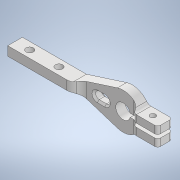
# Autodesk Inventor part: arm_1
Saved by Autodesk Inventor 2020 (Build 240168000, 168)
## iProperties
Created: 2020-01-20
Part Number: arm_1
Material: Generic
Document SubType Name: Modeling
Designer: psrobotics
Density: 1 g/cm^3
Appearance: Default
Author: psrobotics
Autodesk Inventor part; units mm, degrees
ref_plane "YZ Plane" through (0, 0, 0) normal (1, 0, 0) x (0, 1, 0)
ref_plane "XZ Plane" through (0, 0, 0) normal (0, 1, 0) x (-1, 0, 0)
ref_plane "XY Plane" through (0, 0, 0) normal (0, 0, 1) x (1, 0, 0)
sketch "Sketch1" plane through (0, 0, 0) normal (0, 0, 1) x (1, 0, 0)
  circle A0 centre (0, 0) radius 4 projected
  circle A1 centre (0, 0) radius 4
  line L0 (0, 0) -> (-60, 0)
  circle A2 centre (0, 0) radius 10
  line L1 (-60, 0) -> (-60, -2.5)
  line L2 (-60, -2.5) -> (-25, -2.5)
  line L3 (-25, -2.5) -> (-25, 2.5)
  line L4 (-25, 2.5) -> (-60, 2.5)
  line L5 (-60, 2.5) -> (-60, -2.5)
  line L6 (-25, -2.5) -> (-3.0476, -9.5243)
  line L7 (-25, 2.5) -> (-3.0476, 9.5243)
  point P0 (0, 0)
  dimension "d0" = 8
  dimension "d1" = 60
  dimension "d2" = 20
  dimension "d3" = 2.5
  dimension "d4" = 35
  dimension "d5" = 5
  constraints: 16 end point, 2 centre point, 2 coincident, 2 horizontal, 2 parallel, 2 point on circle, 2 tangent, 1 perpendicular, 1 vertical
  measures "d0" diameter of A1
  measures "d1" distance of L0.start L0.end
  measures "d2" diameter of A2
  measures "d3" distance of L0.end L1.end
  measures "d4" distance of L4.end L3.end
  measures "d5" distance of L3.end L2.end
extrude "Extrusion1" add sketch "Sketch1" against normal blind 5
sketch "Sketch2" plane through (0, 0, 0) normal (0, 0, 1) x (1, 0, 0)
  line L0 (-60, 2.5) -> (-60, -2.5) projected
  line L1 (-60, -2.5) -> (-25, -2.5) projected
  line L2 (-25, -2.5) -> (-3.0476, -9.5243) projected
  arc A0 (-3.0476, -9.5243) -> (-3.0476, 9.5243) centre (0, 0) ccw projected
  line L3 (-3.0476, 9.5243) -> (-25, 2.5) projected
  line L4 (-25, 2.5) -> (-60, 2.5) projected
  circle A1 centre (0, 0) radius 4 projected
  line L5 (0, 0) -> (7.6, 0)
  line L6 (13.6, -1) -> (13.6, 1)
  line L7 (13.6, 1) -> (1.6, 1)
  line L8 (1.6, 1) -> (1.6, -1)
  line L9 (1.6, -1) -> (13.6, -1)
  line L10 (13.6, -1) -> (1.6, 1) construction
  line L11 (13.6, 1) -> (1.6, -1) construction
  point P0 (0, 0)
  dimension "d8" = 7.6
  dimension "d9" = 2
  dimension "d10" = 12
  constraints: 14 end point, 2 midpoint, 2 parallel, 2 perpendicular, 1 horizontal
  measures "d8" distance of L5.start L5.end
  measures "d9" distance of L6.start L6.end
  measures "d10" distance of L7.end L6.end
extrude "Extrusion2" cut sketch "Sketch2" against normal blind 5 contours L7 L6 L9 A0 | A0 L9 A1 L7 | A1 L5 L8 L7 | L9 L8 L5 A1
sketch "Sketch3" plane through (0, 0, 0) normal (0, 0, 1) x (1, 0, 0)
  line L0 (3.873, 1) -> (9.9499, 1) projected
  arc A0 (9.9499, 1) -> (-3.0476, 9.5243) centre (0, 0) ccw projected
  line L1 (-3.0476, 9.5243) -> (-25, 2.5) projected
  line L2 (-25, 2.5) -> (-60, 2.5) projected
  line L3 (-60, 2.5) -> (-60, -2.5) projected
  line L4 (-60, -2.5) -> (-25, -2.5) projected
  line L5 (-25, -2.5) -> (-3.0476, -9.5243) projected
  arc A1 (-3.0476, -9.5243) -> (9.9499, -1) centre (0, 0) ccw projected
  line L6 (9.9499, -1) -> (3.873, -1) projected
  arc A2 (3.873, 1) -> (3.873, -1) centre (0, 0) ccw projected
  line L7 (3.873, -1) -> (21.873, -1)
  line L8 (21.873, -1) -> (21.873, -5)
  line L9 (21.873, -5) -> (3.873, -5)
  line L10 (3.873, -5) -> (3.873, -1)
  arc A3 (3.873, 1) -> (3.873, -1) centre (0, 0) ccw projected
  line L11 (3.873, 1) -> (21.873, 1)
  line L12 (21.873, 1) -> (21.873, 5)
  line L13 (21.873, 5) -> (3.873, 5)
  line L14 (3.873, 5) -> (3.873, 1)
  point P0 (0, 0)
  point P1 (9.9499, 1)
  point P2 (9.9499, -1)
  dimension "d13" = 18
  dimension "d14" = 4
  dimension "d15" = 18
  dimension "d16" = 4
  constraints: 16 end point, 4 parallel, 2 horizontal, 2 perpendicular
  measures "d13" distance of L8.end L9.end
  measures "d14" distance of L7.end L8.end
  measures "d15" distance of L13.end L12.end
  measures "d16" distance of L12.end L11.end
extrude "Extrusion3" add sketch "Sketch3" against normal blind 5 contours L14 L13 A0 L0 | A0 L13 L12 L11 | L6 A1 L9 L10 | L7 L8 L9 A1
sketch "Sketch4" plane through (8.6603, 5, 0) normal (0, 1, 0) x (1, 0, 0)
  line L0 (0, 0) -> (0, 5) projected
  line L1 (13.2127, 0) -> (0, 0) projected
  line L2 (13.2127, 0) -> (13.2127, 5) projected
  line L3 (0, 5) -> (13.2127, 5) projected
  line L4 (13.2127, 0) -> (13.2127, 5) projected
  line L5 (13.2127, 5) -> (0, 5)
  line L6 (0, 5) -> (0, -3)
  line L7 (0, -3) -> (13.2127, -3)
  line L8 (13.2127, -3) -> (13.2127, 5)
  point P0 (-8.6603, 0)
  dimension "d19" = 8
  constraints: 8 end point, 2 parallel, 1 horizontal, 1 perpendicular
  measures "d19" distance of L5.end L6.end
extrude "Extrusion4" add sketch "Sketch4" against normal blind 4 contours L1 L8 L7 L6
sketch "Sketch5" plane through (8.6603, -5, 0) normal (0, -1, 0) x (1, 0, 0)
  line L0 (0, 0) -> (0, -5) projected
  line L1 (0, 0) -> (0, 3) projected
  line L2 (0, 3) -> (13.2127, 3) projected
  line L3 (13.2127, 3) -> (13.2127, -5) projected
  line L4 (0, -5) -> (13.2127, -5) projected
  point P0 (-8.6603, 0)
extrude "Extrusion5" add sketch "Sketch5" against normal blind 4
sketch "Sketch6" plane through (8.6603, -5, -5) normal (0, -1, 0) x (1, 0, 0)
  line L0 (0, 0) -> (0, 5) projected
  line L1 (13.2127, 0) -> (0, 0) projected
  line L2 (13.2127, 0) -> (13.2127, 8) projected
  line L3 (13.2127, 8) -> (0, 8) projected
  line L4 (0, 8) -> (0, 5) projected
  line L5 (13.2127, 8) -> (13.2127, 0) projected
  line L6 (13.2127, 4) -> (6.6064, 4)
  circle A0 centre (6.6064, 4) radius 1.5
  point P0 (-8.6603, 5)
  dimension "d24" = 3
  constraints: 2 end point, 1 centre point, 1 coincident, 1 midpoint, 1 perpendicular
  measures "d24" diameter of A0
extrude "Extrusion6" cut sketch "Sketch6" against normal blind 10 contours A0
fillet "Fillet1" radius 3 2 edges at (8.6603, -3, 0) (8.6603, 3, 0)
sketch "Sketch7" plane through (-60, -2.5, 0) normal (0, -1, 0) x (1, 0, 0)
  line L0 (0, 0) -> (35, 0) projected
  line L1 (0, 0) -> (0, -5) projected
  line L2 (35, -5) -> (0, -5) projected
  line L3 (35, 0) -> (35, -5) projected
  line L4 (35, -5) -> (0, -5) projected
  line L5 (0, -5) -> (35, -5)
  line L6 (35, -5) -> (35, 3)
  line L7 (35, 3) -> (0, 3)
  line L8 (0, 3) -> (0, -5)
  point P0 (60, 0)
  dimension "d28" = 35
  dimension "d29" = 8
  constraints: 8 end point, 2 parallel, 1 horizontal, 1 perpendicular
  measures "d28" distance of L7.end L6.end
  measures "d29" distance of L6.end L5.end
extrude "Extrusion7" add sketch "Sketch7" against normal blind 5
fillet "Fillet2" radius 6 1 edges at (-25, 0, 0)
fillet "Fillet3" radius 1.5 4 edges at (21.873, -3, 3) (21.873, 3, 3) (21.873, -3, -5) (21.873, 3, -5)
fillet "Fillet4" radius 3 2 edges at (8.6603, 5, -1) (8.6603, -5, -1)
fillet "Fillet5" radius 2 2 edges at (8.6603, -3.227, 3) (8.6603, 3.227, 3)
sketch "Sketch8" plane through (0, 0, 0) normal (0, 0, 1) x (1, 0, 0)
  line L0 (-19.8038, -4.1627) -> (-19.8038, 4.1627) projected
  line L1 (-19.8038, -4.1627) -> (-3.0476, -9.5243) projected
  arc A0 (-3.0476, -9.5243) -> (5.6603, -8.2439) centre (0, 0) ccw projected
  line L2 (5.6603, -1) -> (5.6603, -8.2439) projected
  line L3 (5.6603, -1) -> (3.873, -1) projected
  arc A1 (3.873, 1) -> (3.873, -1) centre (0, 0) ccw projected
  line L4 (3.873, 1) -> (5.6603, 1) projected
  line L5 (5.6603, 8.2439) -> (5.6603, 1) projected
  arc A2 (5.6603, 8.2439) -> (-3.0476, 9.5243) centre (0, 0) ccw projected
  line L6 (-3.0476, 9.5243) -> (-19.8038, 4.1627) projected
  line L7 (0, 0) -> (-12, 0)
  line L8 (-10, 0) -> (-14, 0) construction
  line L9 (-10, 2) -> (-14, 2)
  line L10 (-14, -2) -> (-10, -2)
  arc A3 (-10, -2) -> (-10, 2) centre (-10, 0) ccw
  arc A4 (-14, 2) -> (-14, -2) centre (-14, 0) ccw
  point P0 (0, 0)
  dimension "d36" = 12
  dimension "d37" = 2
  dimension "d38" = 4
  constraints: 10 end point, 4 point on circle, 4 tangent, 2 centre point, 2 horizontal, 1 midpoint, 1 parallel
  measures "d36" distance of L7.start L7.end
  measures "d37" distance of L7.end L8.end
  measures "d38" diameter of A4
extrude "Extrusion8" cut sketch "Sketch8" against normal blind 5 contours A3 L10 A4 L9
sketch "Sketch9" plane through (-60, -2.5, -5) normal (0, -1, 0) x (1, 0, 0)
  line L0 (0, 8) -> (0, 0) projected
  line L1 (35, 0) -> (0, 0) projected
  line L2 (35, 0) -> (35, 8) projected
  line L3 (35, 8) -> (0, 8) projected
  line L4 (0, 8) -> (0, 0) projected
  line L5 (0, 4) -> (8, 4)
  line L6 (8, 4) -> (24, 4)
  circle A0 centre (24, 4) radius 2
  circle A1 centre (8, 4) radius 2
  point P0 (60, 5)
  dimension "d41" = 8
  dimension "d42" = 16
  dimension "d43" = 4
  dimension "d44" = 4
  constraints: 4 end point, 2 centre point, 2 coincident, 1 horizontal, 1 midpoint, 1 point on line
  measures "d41" distance of L5.start L5.end
  measures "d42" distance of L5.end L6.end
  measures "d43" diameter of A0
  measures "d44" diameter of A1
extrude "Extrusion9" cut sketch "Sketch9" against normal blind 5 contours A1 L6 L5 | L5 L6 A1 | A0
fillet "Fillet6" radius 6 1 edges at (-25, 0, 3)
chamfer "Chamfer1" distance 1 angle 45 8 edges at (-12, -2, 0) (-16, 0, 0) (-12, 2, 0) (-8, 0, 0) (-12, -2, -5) (-8, 0, -5) (-12, 2, -5) (-16, 0, -5)
body "Solid1"
